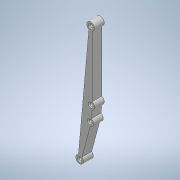
# Autodesk Inventor part: Шаблон2
Saved by Autodesk Inventor 2020 (Build 240168000, 168)
## iProperties
Created: 2021-05-21
Part Number: Шаблон2
Material: Типовые
Document SubType Name: Modeling
Designer: I_Love_U_Bogdan
Density: 1 g/cm^3
Appearance: По умолчанию
Author: I_Love_U_Bogdan
Autodesk Inventor part; units mm, degrees
ref_plane "YZ Plane" through (0, 0, 0) normal (1, 0, 0) x (0, 1, 0)
ref_plane "XZ Plane" through (0, 0, 0) normal (0, 1, 0) x (-1, 0, 0)
ref_plane "XY Plane" through (0, 0, 0) normal (0, 0, 1) x (1, 0, 0)
sketch "Эскиз1" plane through (0, 0, 0) normal (0, 0, 1) x (1, 0, 0)
  circle A0 centre (82.5, -44) radius 1.5 projected
  circle A1 centre (82.5, -114) radius 1.5 projected
  circle A2 centre (81.5042, -129.3151) radius 1.5 projected
  circle A3 centre (71.168, -167.8906) radius 1.5 projected
  line L0 (82.5, -44) -> (82.5, -114) construction
  line L1 (81, -44) -> (81, -114)
  line L2 (84, -114) -> (84, -44)
  arc A4 (84, -44) -> (81, -44) centre (82.5, -44) ccw
  arc A5 (81, -114) -> (84, -114) centre (82.5, -114) ccw
  line L3 (82.5, -114) -> (81.5042, -129.3151) construction
  line L4 (81.0032, -113.9027) -> (80.0074, -129.2178)
  line L5 (83.001, -129.4125) -> (83.9968, -114.0973)
  arc A6 (83.9968, -114.0973) -> (81.0032, -113.9027) centre (82.5, -114) ccw
  arc A7 (80.0074, -129.2178) -> (83.001, -129.4125) centre (81.5042, -129.3151) ccw
  line L6 (81.5042, -129.3151) -> (71.168, -167.8906) construction
  line L7 (80.0553, -128.9269) -> (69.7191, -167.5023)
  line L8 (72.6168, -168.2788) -> (82.9531, -129.7034)
  arc A8 (82.9531, -129.7034) -> (80.0553, -128.9269) centre (81.5042, -129.3151) ccw
  arc A9 (69.7191, -167.5023) -> (72.6168, -168.2788) centre (71.168, -167.8906) ccw
  line L9 (82.5, -44) -> (71.168, -167.8906) construction
  line L10 (81.0062, -43.8634) -> (69.6742, -167.7539)
  line L11 (72.6617, -168.0272) -> (83.9938, -44.1366)
  arc A10 (83.9938, -44.1366) -> (81.0062, -43.8634) centre (82.5, -44) ccw
  arc A11 (69.6742, -167.7539) -> (72.6617, -168.0272) centre (71.168, -167.8906) ccw
  circle A12 centre (82.5, -44) radius 4
  circle A13 centre (82.5, -114) radius 4
  circle A14 centre (81.5042, -129.3151) radius 4
  circle A15 centre (71.168, -167.8906) radius 4
  point P0 (0, 0)
  point P1 (82.5, -79)
  point P2 (82.0021, -121.6576)
  point P3 (76.3361, -148.6029)
  point P4 (76.834, -105.9453)
  point P5 (84, -47.7081)
  point P6 (80.6685, -47.5561)
  point P7 (70.0119, -164.0613)
  point P8 (73.5766, -164.697)
  point P9 (81.9934, -133.2851)
  point P10 (83.2416, -125.7122)
  point P11 (83.7562, -117.7976)
  point P12 (84, -110.2919)
  dimension "d0" = 1.5
  dimension "d1" = 8
  dimension "d2" = 8
  dimension "d3" = 8
  dimension "d4" = 8
  constraints: 32 end point, 16 point on circle, 16 tangent, 12 centre point, 4 coincident, 4 midpoint, 4 parallel, 2 concentric, 1 vertical
  measures "d0" radius of A9
  measures "d1" diameter of A12
  measures "d2" diameter of A13
  measures "d3" diameter of A14
  measures "d4" diameter of A15
extrude "Выдавливание1" add sketch "Эскиз1" along normal blind 10 contours L2 A12 L11 A0 | A0 L10 A12 L2 | A0 L1 A12 L10 | L11 A12 L1 A0 | L2 A13 L1 L11 A12 | A12 L1 L11 L7 A15 L10 | L11 L1 A12 | A13 L5 A1 L2 | L2 A1 L1 A13 | A15 L7 A3 L10 | L10 A3 L8 A15 | L1 A13 L4 A14 L7 L11 | L1 L4 A13 | A15 L11 A3 L7 | L7 L11 A15 | L7 A14 L8 A15 L11 | L5 A13 L4 A1 | L5 A14 L4 A13 | A3 L11 A15 L8 | A14 L4 L7 | L7 L4 A2 L8 A14 | A14 L8 A2 L5 | L5 A2 L7 L4 A14 | L7 A2 L4
chamfer "Фаска1" distance 1 angle 45 8 edges at (81, -44, 10) (81, -114, 10) (80.0042, -129.3151, 10) (69.668, -167.8906, 10) (80.0042, -129.3151, 0) (81, -114, 0) (81, -44, 0) (69.668, -167.8906, 0)
